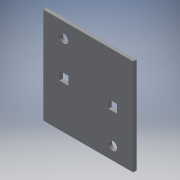
# Autodesk Inventor part: Platine
Saved by Autodesk Inventor 2019 (Build 230136000, 136)
## iProperties
Created: 2022-10-31
Part Number: Platine
Material: Generisch
Document SubType Name: Modeling
Designer: RP
Density: 1 g/cm^3
Appearance: Glatt - waldgrün
Author: RP
Autodesk Inventor part; units mm, degrees
ref_plane "YZ Plane" through (0, 0, 0) normal (1, 0, 0) x (0, 1, 0)
ref_plane "XZ Plane" through (0, 0, 0) normal (0, 1, 0) x (-1, 0, 0)
ref_plane "XY Plane" through (0, 0, 0) normal (0, 0, 1) x (1, 0, 0)
sketch "Skizze1" plane through (0, 0, 0) normal (0, 0, 1) x (1, 0, 0)
  line L0 (21, 24.1) -> (-21, 24.1)
  line L1 (-21, 24.1) -> (-21, -21.2)
  line L2 (-21, -21.2) -> (21, -21.2)
  line L3 (21, -21.2) -> (21, 24.1)
  line L4 (10.45, 2) -> (14.55, 2)
  line L5 (14.55, 2) -> (14.55, -2)
  line L6 (14.55, -2) -> (10.45, -2)
  line L7 (10.45, -2) -> (10.45, 2)
  circle A0 centre (12.5, -16) radius 2
  circle A1 centre (-12.5, 16) radius 2
  line L8 (-10.45, 2) -> (-14.55, 2)
  line L9 (-14.55, 2) -> (-14.55, -2)
  line L10 (-14.55, -2) -> (-10.45, -2)
  line L11 (-10.45, -2) -> (-10.45, 2)
  line L12 (12.5, 2) -> (12.5, -2) construction
  line L13 (-12.5, 2) -> (-12.5, -2) construction
  line L14 (14.55, 0) -> (-14.55, 0) construction
  line L15 (0, 0) -> (0, 31.6148) construction
  dimension "d1" = 42
  dimension "d3" = 4
  dimension "d4" = 4
  dimension "d5" = 16
  dimension "d6" = 16
  dimension "d7" = 4
  dimension "d8" = 4.1
  dimension "d9" = 21.2
  dimension "d12" = 25
  dimension "d13" = 24.1
  constraints: 32 end point, 7 midpoint, 6 parallel, 3 horizontal, 3 perpendicular, 2 centre point, 2 collinear, 2 point on line, 1 coincident, 1 vertical, 2 other
  measures "d1" distance of L0.start L0.end
  measures "d3" diameter of A1
  measures "d4" diameter of A0
  measures "d5" distance from line of L14 A1.centre
  measures "d6" distance from line of A0.centre L14
  measures "d7" distance of L8.end L9.end
  measures "d8" distance of L8.start L8.end
  measures "d9" distance between parallel lines of L2 L14
  measures "d12" distance between parallel lines of L12 L13
  measures "d13" distance between parallel lines of L0 L14
extrude "Extrusion1" add sketch "Skizze1" along normal blind 1.6
